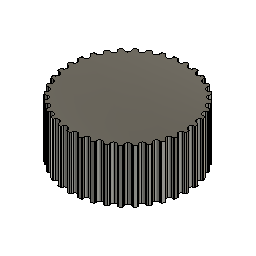
gear_36z (Autodesk Fusion 360 design; units mm, degrees)
Autodesk Fusion 360 part; units mm, degrees
sketch "Sketch1" plane through (0, 0, 0) normal (0, 0, 1) x (1, 0, 0) in component "gt2 pulley"
  circle A0 centre (0, 0) radius 11.4592 construction
  circle A1 centre (0, 0) radius 10.4552 construction
  line L0 (0, 0) -> (0, 11.4592) construction
  line L1 (0, 0) -> (0.9987, 11.4156) construction
  line L2 (0, 0) -> (1.4091, 11.3722) construction
  circle A2 centre (0, 0) radius 11.2052 construction
  arc A3 (0.3796, 11.0616) -> (0.4379, 10.7789) centre (1.3779, 11.1201) ccw
  circle A4 centre (0, 0) radius 11.0552 construction
  arc A5 (0.2329, 11.2027) -> (0, 11.2052) centre (0, 0) ccw
  arc A6 (0.3796, 11.0616) -> (0.2329, 11.2027) centre (0.2299, 11.0528) ccw
  arc A7 (0.4379, 10.7789) -> (0.9112, 10.4154) centre (0.9596, 10.9683) ccw
  arc A8 (0, 11.2052) -> (-0.2329, 11.2027) centre (0, 0) ccw
  arc A9 (-0.2329, 11.2027) -> (-0.3796, 11.0616) centre (-0.2299, 11.0528) ccw
  arc A10 (-0.4379, 10.7789) -> (-0.3796, 11.0616) centre (-1.3779, 11.1201) ccw
  arc A11 (-0.9112, 10.4154) -> (-0.4379, 10.7789) centre (-0.9596, 10.9683) ccw
  arc A12 (0.9112, 10.4154) -> (-0.9112, 10.4154) centre (0, 0) ccw
  point P0 (1.3779, 11.1201)
  point P1 (0, 11.2052)
  dimension "d18" = 22.9183
  dimension "d19" = 5
  dimension "d22" = 1.004
  dimension "d24" = 0.75
  dimension "d26" = 1
  dimension "d27" = 0.15
  dimension "d28" = 0.15
  dimension "d47" = 0.555
  dimension "d52" = 3.812
  constraint coincident A0.centre A1.centre
  constraint coincident A0 L0.end
  constraint vertical L0
  constraint coincident A0 L1.end
  constraint coincident A0 L2.end
  constraint concentric A1 A2
  constraint coincident A1 A7.end
  constraint coincident L1 A7.end
  constraint coincident A2 P0
  constraint coincident L2 P0
  constraint coincident P0 A3.centre
  constraint coincident A2 P1
  constraint coincident L0 P1
  constraint concentric A2 A4
  constraint coincident P1 A5.end
  constraint coincident A4 A6.centre
  constraint coincident A3.start A6.start
  constraint tangent A3 A6
  constraint tangent A3 A7
  constraint symmetric L0 A7.end A11.start
  constraint symmetric L0 A3.start A9.end
  constraint symmetric L0 A3.end A10.start
  constraint symmetric L0 A3 A10
  constraint symmetric L0 A5.start A8.end
  constraint symmetric L0 P1 A5.end
  constraint symmetric L0 A5 A8
  constraint symmetric L0 A6 A9
  constraint symmetric L0 A7 A11
  constraint coincident A1 A11.start
  constraint tangent A1 A7
  constraint coincident L1 A7.centre
  measures "d18" diameter of A0
  measures "d19" angle of L0 L1
  measures "d22" distance of A0 A1
  measures "d24" distance of A1 A2
  measures "d26" radius of A3
  measures "d27" distance of A2 A4
  measures "d28" radius of A6
  measures "d47" radius of A7
extrude "Extrude1" add sketch "Sketch1" along normal blind 10 makes body 1
pattern_circular "C-Pattern1" count 36 over 360 about axis through (0, 0, 1.75) along (0, 0, 1) of bodies 1 makes body 2 at (-1.113, 10.3957, 3.3333) makes body 3 at (-4.234, 9.5595, 6.6667) makes body 4 at (-5.8296, 8.679, 6.6667) makes body 5 at (-6.7978, 7.9436, 6.6667) makes body 6 at (-8.4465, 6.1618, 6.6667) makes body 7 at (-9.3881, 4.6015, 6.6667) makes body 8 at (-10.0445, 2.9013, 6.6667) makes body 9 at (-10.1495, 2.5097, 3.3333) makes body 10 at (-10.4311, -0.7091, 6.6667) makes body 11 at (-10.1495, -2.5097, 6.6667) makes body 12 at (-9.5595, -4.234, 6.6667) makes body 13 at (-8.679, -5.8296, 6.6667) makes body 14 at (-7.9436, -6.7978, 6.6667) makes body 15 at (-6.1618, -8.4465, 6.6667) makes body 16 at (-4.6015, -9.3881, 6.6667) makes body 17 at (-3.4804, -9.8588, 6.6667) makes body 18 at (-1.113, -10.3957, 6.6667) makes body 19 at (0.7091, -10.4311, 6.6667) makes body 20 at (1.113, -10.3957, 3.3333) makes body 21 at (4.234, -9.5595, 6.6667) makes body 22 at (5.8296, -8.679, 6.6667) makes body 23 at (6.7978, -7.9436, 6.6667) makes body 24 at (8.4465, -6.1618, 6.6667) makes body 25 at (9.1047, -5.1395, 6.6667) makes body 26 at (9.8588, -3.4804, 6.6667) makes body 27 at (10.3957, -1.113, 6.6667) makes body 28 at (10.4311, 0.7091, 6.6667) makes body 29 at (10.1495, 2.5097, 6.6667) makes body 30 at (9.5595, 4.234, 6.6667) makes body 31 at (8.679, 5.8296, 6.6667) makes body 32 at (7.9436, 6.7978, 6.6667) makes body 33 at (7.2482, 7.5349, 3.3333) makes body 34 at (5.1395, 9.1047, 6.6667) makes body 35 at (2.9013, 10.0445, 6.6667) makes body 36 at (1.113, 10.3957, 6.6667)
sketch "Sketch2" plane through (0, 0, 10) normal (0, 0, 1) x (-1, 0, 0)
  arc A0 (-9.7694, -5.202) -> (-9.8183, -5.3997) centre (-9.6869, -5.3273) ccw
  arc A1 (-9.8183, -5.3997) -> (-9.5854, -5.8031) centre (0, 0) ccw
  arc A2 (-9.5854, -5.8031) -> (-9.3898, -5.8595) centre (-9.457, -5.7254) ccw
  arc A3 (-9.1158, -5.7687) -> (-9.3898, -5.8595) centre (-8.9414, -6.7533) ccw
  arc A4 (-8.5644, -5.9968) -> (-9.1158, -5.7687) centre (-9.019, -6.3152) ccw
  arc A5 (-9.4756, -4.4185) -> (-8.5644, -5.9968) centre (0, 0) ccw
  arc A6 (-9.5537, -5.0102) -> (-9.4756, -4.4185) centre (-9.9786, -4.6531) ccw
  arc A7 (-9.7694, -5.202) -> (-9.5537, -5.0102) centre (-10.3192, -4.3668) ccw
  circle A8 centre (0, 0) radius 10.4552
  constraint concentric A1 A8
extrude "Extrude2" add sketch "Sketch2" against normal blind 10 contours A5 A8 bodies 1 2 3 4 5 6 7 8 9 10 11 12 13 14 15 16 17 18 19 20 21 22 23 24 25 26 27 28 29 30 31 32 33 34 35 36
extrude "Extrude4" [suppressed] in component "gt2 pulley"
pattern_circular "C-Pattern7" [suppressed] in component "gt2 pulley"
extrude "Extrude3" [suppressed] in component "gt2 pulley"
pattern_circular "C-Pattern6" [suppressed] in component "gt2 pulley"
extrude "Extrude2'" [suppressed] in component "gt2 pulley"
pattern_circular "C-Pattern5" [suppressed] in component "gt2 pulley"
extrude "Extrude1'" [suppressed] in component "gt2 pulley"
pattern_circular "C-Pattern4" [suppressed] in component "gt2 pulley"
pattern_circular "C-Pattern3" [suppressed] in component "gt2 pulley"
pattern_circular "C-Pattern2" [suppressed] in component "gt2 pulley"
pattern_circular "C-Pattern1'" [suppressed] in component "gt2 pulley"
copy_body "Body->Comp1" [suppressed] in component "Component"
copy_body "Body->Comp2" [suppressed] in component "Component'"
copy_body "Body->Comp3" [suppressed] in component "Component''"
copy_body "Body->Comp4" [suppressed] in component "Component'''"
copy_body "Body->Comp5" [suppressed] in component "Component''''"
copy_body "Body->Comp6" [suppressed] in component "Component'''''"
copy_body "Body->Comp7" [suppressed] in component "Component''''''"
copy_body "Body->Comp8" [suppressed] in component "Component'''''''"
copy_body "Body->Comp9" [suppressed] in component "Component''''''''"
copy_body "Body->Comp10" [suppressed] in component "Component'''''''''"
copy_body "Body->Comp11" [suppressed] in component "Component''''''''''"
copy_body "Body->Comp12" [suppressed] in component "Component'''''''''''"
copy_body "Body->Comp13" [suppressed] in component "Component''''''''''''"
copy_body "Body->Comp14" [suppressed] in component "Component'''''''''''''"
copy_body "Body->Comp15" [suppressed] in component "Component''''''''''''''"
copy_body "Body->Comp16" [suppressed] in component "Component'''''''''''''''"
copy_body "Body->Comp17" [suppressed] in component "Component''''''''''''''''"
copy_body "Body->Comp18" [suppressed] in component "Component'''''''''''''''''"
copy_body "Body->Comp19" [suppressed] in component "Component''''''''''''''''''"
copy_body "Body->Comp20" [suppressed] in component "Component'''''''''''''''''''"
component "gt2 pulley" placed x (1, 0, 0) y (0, 1, 0) z (0, 0, 1) at (0, 0, 0)
equation "NumTeeth = 36" comment "min 20"
equation "ToothPitch = 2 mm"
equation "PullyDia = NumTeeth * ToothPitch / PI"
equation "ToothAng = ( ( 360 / NumTeeth ) * 1 deg )"
equation "TransOffsetAngle = ToothAng * 0.2"
equation "Sholulder_Radius = 0.15 mm"
equation "Root_Radius = 0.555 mm"
equation "TransRadius = 1 mm"
equation "ToolHeight = 0.75 mm"
equation "PLD = 0.254 mm"
equation "d18 = PullyDia"
equation "d19 = ToothAng / 2"
equation "d22 = PLD + ToolHeight"
equation "d24 = ToolHeight"
equation "d26 = TransRadius"
equation "d27 = Sholulder_Radius"
equation "d31 = NumTeeth"
equation "d33 = NumTeeth"
equation "d35 = NumTeeth"
equation "d37 = NumTeeth"
equation "d41 = NumTeeth"
equation "d45 = NumTeeth"
equation "d47 = Root_Radius"
equation "d50 = NumTeeth"
